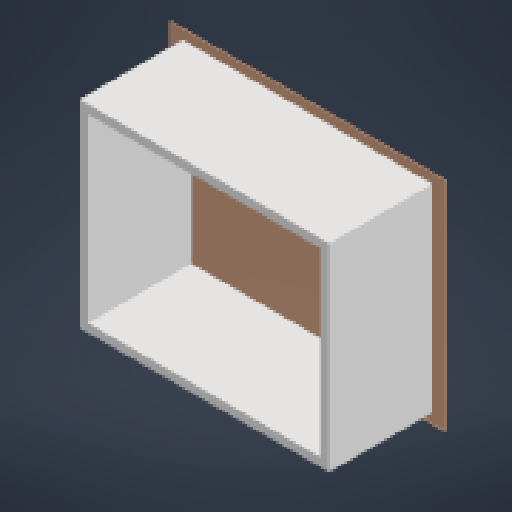
# Autodesk Inventor part: schale
Saved by Autodesk Inventor 2027 (Build 310192060, 192F)
## iProperties
Created: 2026-06-17
Part Number: schale
Material: Generic
Document SubType Name: Modeling
Designer: Felix
Density: 1 g/cm^3
Appearance: Default
Author: Felix
Autodesk Inventor part; units mm, degrees
ref_plane "YZ Plane" through (0, 0, 0) normal (1, 0, 0) x (0, 1, 0)
ref_plane "XZ Plane" through (0, 0, 0) normal (0, 1, 0) x (-1, 0, 0)
ref_plane "XY Plane" through (0, 0, 0) normal (0, 0, 1) x (1, 0, 0)
ref_plane "Work Plane1" through (0, 0, 0) normal (0, 0, 1) x (1, 0, 0)
ref_plane "Work Plane2" through (0, 0, 0) normal (0, 0, 1) x (1, 0, 0)
ref_plane "Work Plane3" through (0, 0, 0) normal (0, 0, 1) x (1, 0, 0)
sketch "Sketch2" plane through (0, 0, 0) normal (0, 0, 1) x (1, 0, 0)
  circle A0 centre (-67.5, -52.5) radius 1.75 projected
  circle A1 centre (67.5, -52.5) radius 1.75 projected
  circle A2 centre (-67.5, 52.5) radius 1.75 projected
  circle A3 centre (67.5, 52.5) radius 1.75 projected
  circle A4 centre (52.5, 37.5) radius 2 projected
  circle A5 centre (10.5, -14.5) radius 2 projected
  circle A6 centre (-24.5, -0.6) radius 2 projected
  circle A7 centre (52.5, 5.5) radius 2 projected
  circle A8 centre (-5.5, 37.5) radius 2 projected
  circle A9 centre (-24.5, -37.5) radius 2 projected
  circle A10 centre (57.5, -14.5) radius 2 projected
  circle A11 centre (57.5, -37.5) radius 2 projected
  circle A12 centre (-61.4, -0.6) radius 2 projected
  line L0 (-72.5, -57.5) -> (-72.5, 57.5) projected
  line L1 (72.5, -57.5) -> (-72.5, -57.5) projected
  line L2 (72.5, 57.5) -> (72.5, -57.5) projected
  line L3 (-72.5, 57.5) -> (72.5, 57.5) projected
  line L4 (67.5, 52.5) -> (67.5, -52.5)
  line L5 (67.5, -52.5) -> (-67.5, -52.5)
  line L6 (-67.5, -52.5) -> (-67.5, 52.5)
  line L7 (-67.5, 52.5) -> (67.5, 52.5)
  point P0 (0, 0)
  dimension "d3" = 5
  constraints: 8 end point, 3 other
  measures "d3" distance between parallel lines of L3 L7
extrude "Extrusion1" add sketch "Sketch2" along normal blind 60 contours A0 L6 L5 | L5 L4 A1 | A2 L7 L6 | L4 L7 A3 | L0 L3 L2 L1 picked at (-67.8303, -53.6096) picked at (66.3503, -52.6396) picked at (-67.9208, 51.4215) picked at (67.2228, 53.6245)
sketch "Sketch3" plane through (0, 0, 60) normal (0, 0, 1) x (1, 0, 0)
  line L0 (-72.5, 57.5) -> (-72.5, -57.5) projected
  line L1 (-72.5, 57.5) -> (72.5, 57.5)
  line L2 (72.5, 57.5) -> (72.5, -57.5)
  line L3 (72.5, -57.5) -> (-72.5, -57.5)
  line L4 (-72.5, -57.5) -> (-72.5, 57.5)
  point P0 (0, 0)
  constraints: 8 end point, 2 parallel, 1 horizontal, 1 perpendicular
extrude "Extrusion2" add sketch "Sketch3" along normal blind 5
sketch "Sketch4" plane through (72.5, -57.5, 0) normal (1, 0, 0) x (0, 0, -1)
  line L0 (-16.25, 27.75) -> (-16.25, 35.25) construction
  line L1 (-20, 27.75) -> (-20, 35.25)
  line L2 (-12.5, 35.25) -> (-12.5, 27.75)
  arc A0 (-20, 27.75) -> (-12.5, 27.75) centre (-16.25, 27.75) ccw
  arc A1 (-12.5, 35.25) -> (-20, 35.25) centre (-16.25, 35.25) ccw
  line L3 (0, 0) -> (0, 115) projected
  line L4 (5.7, 18) -> (5.7, 22) projected
  line L5 (0, 115) -> (0, 0) projected
  line L6 (0, 0) -> (10, 0) projected
  line L7 (10, 115) -> (10, 0) projected
  line L8 (0, 115) -> (10, 115) projected
  line L9 (0, 41) -> (5.7, 41)
  line L10 (0, 22) -> (5.7, 22)
  circle A2 centre (-40, 31.5) radius 5
  point P0 (0, 57.5)
  point P1 (-16.25, 31.5)
  point P2 (-20, 31.5)
  point P3 (-16.25, 24)
  point P4 (-16.25, 39)
  point P5 (5.7, 20)
  dimension "d8" = 20
  dimension "d9" = 7.5
  dimension "d10" = 15
  dimension "d12" = 9.5
  dimension "d13" = 10
  dimension "d14" = 20
  dimension "d15" = 0
  constraints: 12 end point, 6 point on circle, 4 tangent, 3 centre point, 3 midpoint, 2 horizontal, 1 parallel, 1 vertical, 3 other
  measures "d8" distance from line of L3 point (-20, 31.5)
  measures "d9" distance between parallel lines of L1 L2
  measures "d10" distance of point (-16.25, 24) point (-16.25, 39)
  measures "d12" distance from line of L10 point (-16.25, 31.5)
  measures "d13" diameter of A2
  measures "d14" distance from line of L1 A2.centre
  measures "d15" vertical distance of point (-20, 31.5) A2.centre
extrude "Extrusion3" cut sketch "Sketch4" against normal up to next contours L1 A1 L2 A0 | A2
sketch "Sketch5" plane through (-72.5, -57.5, 0) normal (-1, 0, 0) x (0, 0, 1)
  circle A0 centre (40, 90) radius 12.2
  line L0 (65, 115) -> (65, 0) projected
  line L1 (0, 115) -> (65, 115) projected
  point P0 (0, 57.5)
  dimension "d18" = 24.4
  dimension "d19" = 25
  dimension "d20" = 25
  constraints: 1 centre point
  measures "d18" diameter of A0
  measures "d19" distance from line of L0 A0.centre
  measures "d20" distance from line of L1 A0.centre
extrude "Extrusion4" cut sketch "Sketch5" against normal blind 10
sketch "Sketch6" plane through (-67.5, -52.5, 0) normal (1, 0, 0) x (0, 0, -1)
  circle A0 centre (-40, 85) radius 12.2 projected
  circle A1 centre (-40, 85) radius 17.5
  point P0 (0, 52.5)
  dimension "d23" = 35
  constraints: 1 centre point, 1 coincident
  measures "d23" diameter of A1
extrude "Extrusion5" add sketch "Sketch6" along normal blind 8
sketch "Sketch8" plane through (0, 0, 0) normal (0, 0, -1) x (-1, 0, 0)
  line L0 (72.5, -57.5) -> (-72.5, -57.5) projected
  line L1 (72.5, -57.5) -> (62.5, -57.5)
  line L2 (62.5, -57.5) -> (62.5, -47.5)
  line L3 (62.5, -47.5) -> (72.5, -47.5)
  line L4 (72.5, -47.5) -> (72.5, -57.5)
  line L5 (0, -57.5) -> (0, 57.5)
  line L6 (-72.5, 57.5) -> (72.5, 57.5) projected
  line L7 (72.5, 57.5) -> (72.5, -57.5) projected
  line L8 (72.5, 0) -> (-72.5, 0)
  line L9 (-72.5, -57.5) -> (-62.5, -57.5)
  line L10 (-62.5, -57.5) -> (-62.5, -47.5)
  line L11 (-62.5, -47.5) -> (-72.5, -47.5)
  line L12 (-72.5, -47.5) -> (-72.5, -57.5)
  line L13 (72.5, 57.5) -> (62.5, 57.5)
  line L14 (62.5, 57.5) -> (62.5, 47.5)
  line L15 (62.5, 47.5) -> (72.5, 47.5)
  line L16 (72.5, 47.5) -> (72.5, 57.5)
  line L17 (-72.5, 57.5) -> (-62.5, 57.5)
  line L18 (-62.5, 57.5) -> (-62.5, 47.5)
  line L19 (-62.5, 47.5) -> (-72.5, 47.5)
  line L20 (-72.5, 47.5) -> (-72.5, 57.5)
  circle A0 centre (67.5, -52.5) radius 2
  circle A1 centre (67.5, 52.5) radius 2
  circle A2 centre (-67.5, -52.5) radius 2
  circle A3 centre (-67.5, 52.5) radius 2
  point P0 (0, 0)
  dimension "d31" = 10
  dimension "d32" = 10
  dimension "d35" = 4
  dimension "d36" = 5
  dimension "d37" = 5
  constraints: 36 end point, 12 symmetric about line, 4 centre point, 3 midpoint, 2 horizontal, 2 parallel, 1 perpendicular, 3 other
  measures "d31" distance between parallel lines of L0 L3
  measures "d32" distance between parallel lines of L4 L2
  measures "d35" diameter of A0
  measures "d36" distance from line of L3 A0.centre
  measures "d37" distance from line of L2 A0.centre
extrude "Extrusion7" add sketch "Sketch8" against normal blind 10 contours L0 L2 L3 L4 | L15 L14 L6 L7 | L0 L12 L11 L10 | L6 L18 L19 L20 | A0 | A1 | A2 | A3
sketch "Sketch9" plane through (0, 0, 0) normal (0, 0, -1) x (-1, 0, 0)
  circle A0 centre (-67.5, -52.5) radius 2
  line L0 (-72.5, -57.5) -> (-72.5, 57.5) projected
  line L1 (-62.5, -47.5) -> (-67.5, -47.5) projected
  line L2 (-72.5, 0) -> (72.5, 0)
  line L3 (72.5, 57.5) -> (72.5, -57.5) projected
  line L4 (-62.5, -52.5) -> (62.5, -52.5) projected
  line L5 (0, -52.5) -> (0, 52.5)
  line L6 (62.5, 52.5) -> (-62.5, 52.5) projected
  circle A1 centre (-67.5, 52.5) radius 2
  circle A2 centre (67.5, -52.5) radius 2
  circle A3 centre (67.5, 52.5) radius 2
  point P0 (0, 0)
  dimension "d38" = 5
  dimension "d39" = 5
  dimension "d40" = 4
  constraints: 4 centre point, 4 end point, 4 midpoint, 3 symmetric about line, 3 other
  measures "d38" distance from line of L0 A0.centre
  measures "d39" distance from line of L1 A0.centre
  measures "d40" diameter of A0
extrude "Extrusion8" cut sketch "Sketch9" against normal blind 5.7
sketch "Sketch10" plane through (-67.5, -52.5, 60) normal (1, 0, 0) x (0, 0, -1)
  line L0 (50, 100) -> (50, 105) projected
  line L1 (50, 105) -> (0, 105) projected
  line L2 (0, 0) -> (0, 105) projected
  line L3 (50, 0) -> (0, 0) projected
  line L4 (50, 0) -> (50, 5) projected
  line L5 (50, 5) -> (60, 5) projected
  line L6 (60, 5) -> (60, 100) projected
  line L7 (60, 100) -> (50, 100) projected
  circle A0 centre (20, 85) radius 17.5 projected
  line L8 (20, 67.5) -> (0, 67.5)
  circle A1 centre (20, 85) radius 17.5 projected
  line L9 (37.5, 85) -> (37.5, 105)
  point P0 (60, 52.5)
  constraints: 4 end point, 2 perpendicular, 2 point on line, 1 horizontal, 1 point on circle, 1 tangent, 2 other
extrude "Extrusion9" add sketch "Sketch10" along normal blind 8 contours L9 A0 L8 L2 L1
sketch "Sketch7" plane through (0, 0, 0) normal (0, 0, -1) x (-1, 0, 0)
  line L0 (59.5, 50) -> (59.5, 15) projected
  line L1 (67.5, 15) -> (67.5, 50) projected
  circle A0 centre (63.5, 32.5) radius 1.6
  point P0 (0, 0)
  dimension "d26" = 17.5
  dimension "d27" = 4
  dimension "d28" = 3.2
  constraints: 1 centre point
  measures "d26" vertical distance of L1.start A0.centre
  measures "d27" distance from line of L0 A0.centre
  measures "d28" diameter of A0
extrude "Extrusion6" cut sketch "Sketch7" against normal blind 40
chamfer "Chamfer1" distance 5 angle 60 1 edges at (-65, -47.5, 10) measured on face at (-65, -48, 10)
chamfer "Chamfer2" distance 5 angle 60 1 edges at (-65, 47.5, 10) measured on face at (-65, 48, 10)
chamfer "Chamfer3" distance 5 angle 60 1 edges at (65, 47.5, 10) measured on face at (65, 48, 10)
chamfer "Chamfer4" distance 5 angle 60 1 edges at (65, -47.5, 10) measured on face at (65, -48, 10)
body "Solid1"
